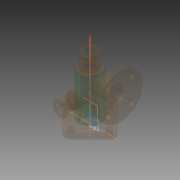
# Autodesk Inventor part: Piesa 3 3D
Saved by Autodesk Inventor 2011 SP2 (Build 150309200, 309)
## iProperties
Created: 2023-03-13
Part Number: Piesa 3 3D
Document SubType Name: Modeling
Designer: utilizator
Density: 1 g/cm^3
Author: utilizator
Autodesk Inventor part; units mm, degrees
ref_plane "XY Plane" through (0, 0, 0) normal (0, 0, 1) x (1, 0, 0)
sketch "Sketch1" plane through (0, 0, 0) normal (0, 0, 1) x (1, 0, 0)
  line L0 (-69.2965, 0) -> (69.2965, 0) projected
  line L1 (0, -69.2965) -> (0, 69.2965) projected
  line L2 (42.4264, -7.0711) -> (7.0711, -42.4264)
  line L3 (-7.0711, -42.4264) -> (-42.4264, -7.0711)
  line L4 (-42.4264, 7.0711) -> (-7.0711, 42.4264)
  line L5 (7.0711, 42.4264) -> (42.4264, 7.0711)
  arc A0 (7.0711, 42.4264) -> (-7.0711, 42.4264) centre (0, 35.3553) ccw
  arc A1 (42.4264, -7.0711) -> (42.4264, 7.0711) centre (35.3553, 0) ccw
  arc A2 (-7.0711, -42.4264) -> (7.0711, -42.4264) centre (0, -35.3553) ccw
  arc A3 (-42.4264, 7.0711) -> (-42.4264, -7.0711) centre (-35.3553, 0) ccw
  circle A4 centre (0, 35) radius 5
  circle A5 centre (35, 0) radius 5
  circle A6 centre (0, -35) radius 5
  circle A7 centre (-35, 0) radius 5
  point P0 (0, 0)
  point P1 (0, 0)
  point P2 (49.4975, 0)
  point P3 (0, -49.4975)
  point P4 (-49.4975, 0)
  point P5 (0, 49.4975)
  point P6 (0, 0)
  point P7 (0, 0)
  point P8 (0, -49.4975)
  point P9 (0, 0)
  point P10 (0, 0)
  point P11 (-49.4975, 0)
  point P12 (0, 0)
  point P13 (0, 0)
  point P14 (0, 49.4975)
  dimension "d0" = 70
  dimension "d1" = 10
  dimension "d2" = 10
  dimension "d3" = 10
  dimension "d4" = 10
  dimension "d5" = 5
  dimension "d6" = 35
  dimension "d9" = 360
  constraints: 10 point on line, 8 centre point, 8 end point, 8 point on circle, 8 tangent, 6 coincident, 1 vertical alignment, 27 other
  measures "d0" distance of point (0, 49.497) point (49.497, 0)
  measures "d1" radius of A0
  measures "d2" radius of A1
  measures "d3" radius of A2
  measures "d4" radius of A3
  measures "d5" radius of A4
  measures "d6" distance of point (0, 0) A4.centre
extrude "Extrusion1" add sketch "Sketch1" along normal blind 10 contours A3 L4 A0 L1 A4 L0 A7 | L0 A7 L1 A6 A2 L3 A3 | L1 A4 A0 L5 A1 L0 A5 | L0 A5 A1 L2 A2 L1 A6
sketch "Sketch2" plane through (0, 0, 10) normal (0, 0, 1) x (1, 0, 0)
  circle A0 centre (0, 0) radius 20
  dimension "d13" = 20
  constraints: 1 centre point, 1 coincident
  measures "d13" radius of A0
extrude "Extrusion2" add sketch "Sketch2" along normal blind 80 separate body
sketch "Sketch3" plane through (0, 0, 90) normal (0, 0, 1) x (1, 0, 0)
  circle A0 centre (0, 0) radius 20 projected
  circle A1 centre (0, 0) radius 15
  dimension "d16" = 15
  constraints: 1 centre point, 1 coincident
  measures "d16" radius of A1
extrude "Extrusion3" add sketch "Sketch3" along normal blind 25 separate body contours A1
ref_plane "Work Plane1" through (0, -55, 0) normal (0, 1, 0) x (-1, 0, 0)
sketch "Sketch4" plane through (0, -55, 0) normal (0, 1, 0) x (-1, 0, 0)
  circle A0 centre (0, 50) radius 13.5
  point P0 (0, 0)
  dimension "d20" = 13.5
  dimension "d21" = 50
  constraints: 1 centre point, 1 vertical alignment
  measures "d20" radius of A0
  measures "d21" distance of point (0, 0) A0.centre
extrude "Extrusion4" add sketch "Sketch4" along normal blind 24 separate body
sketch "Sketch5" plane through (0, -31, 50) normal (0, 1, 0) x (1, 0, 0)
  circle A0 centre (0, 0) radius 13.5 projected
  circle A1 centre (0, 0) radius 13
  point P0 (0, 50)
  dimension "d24" = 13
  constraints: 1 centre point, 1 coincident
  measures "d24" radius of A1
extrude "Extrusion5" add sketch "Sketch5" along normal blind 3 separate body contours A1
sketch "Sketch6" plane through (0, -28, 50) normal (0, 1, 0) x (1, 0, 0)
  circle A0 centre (0, 0) radius 13 projected
  circle A1 centre (0, 0) radius 15
  point P0 (0, 50)
  dimension "d27" = 15
  constraints: 1 centre point, 1 coincident
  measures "d27" radius of A1
extrude "Extrusion6" add sketch "Sketch6" along normal up to surface separate body contours A0 | A1 round surface about axis through (0, 0, 10) along (0, 0, 1) radius 20 far side no
ref_plane "Work Plane2" through (55, 0, 0) normal (1, 0, 0) x (0, 1, 0)
sketch "Sketch7" plane through (55, 0, 0) normal (1, 0, 0) x (0, 1, 0)
  circle A0 centre (0, 70) radius 40
  circle A1 centre (21.2132, 91.2132) radius 5
  circle A2 centre (21.2132, 48.7868) radius 5
  circle A3 centre (-21.2132, 48.7868) radius 5
  circle A4 centre (-21.2132, 91.2132) radius 5
  point P0 (0, 0)
  point P1 (25.813, 70)
  point P2 (0, 44.187)
  point P3 (-25.813, 70)
  point P4 (0, 95.813)
  dimension "d31" = 40
  dimension "d32" = 70
  dimension "d33" = 5
  dimension "d34" = 30
  dimension "d35" = 45
  dimension "d38" = 360
  constraints: 5 centre point, 2 coincident, 1 horizontal alignment, 1 vertical alignment, 14 other
  measures "d31" radius of A0
  measures "d32" distance of point (0, 0) A0.centre
  measures "d33" radius of A1
  measures "d34" distance of A0.centre A1.centre
extrude "Extrusion7" add sketch "Sketch7" against normal blind 10 separate body
sketch "Sketch8" plane through (45, 0, 70) normal (-1, 0, 0) x (0, 0, 1)
  circle A0 centre (0, 0) radius 40 projected
  circle A1 centre (0, 0) radius 15
  point P0 (-70, 0)
  dimension "d42" = 15
  constraints: 1 centre point, 1 coincident
  measures "d42" radius of A1
extrude "Extrusion8" add sketch "Sketch8" along normal up to surface separate body contours A1 round surface about axis through (0, 0, 10) along (0, 0, 1) radius 20 far side no
hole "Hole3" at (0, 0, 115) direction (0, 0, -1) diameter 16 depth 30 bodies 3 2
hole "Hole4" at (0, 0, 85) direction (0, 0, -1) diameter 25 depth 50 bodies 2
sketch "Sketch10" plane through (0, 0, 0) normal (0, 1, 0) x (-1, 0, 0)
  line L0 (0, -23) -> (0, 138) projected
  line L1 (12.5, 35) -> (-12.5, 35) projected
  line L2 (40, 0) -> (30, 0) projected
  line L3 (5, 0) -> (-5, 0) projected
  line L4 (-30, 0) -> (-40, 0) projected
  line L5 (5, 0) -> (-5, 0) projected
  line L6 (7.0711, 0) -> (42.4264, 0) projected
  line L7 (-7.0711, 0) -> (7.0711, 0) projected
  line L8 (-42.4264, 0) -> (-7.0711, 0) projected
  line L9 (-42.4264, 0) -> (-42.4264, 0) projected
  line L10 (-7.0711, 0) -> (-42.4264, 0) projected
  line L11 (7.0711, 0) -> (-7.0711, 0) projected
  line L12 (42.4264, 0) -> (7.0711, 0) projected
  line L13 (42.4264, 0) -> (42.4264, 0) projected
  line L14 (-12.5, 35) -> (-15, 0)
  line L15 (-15, 0) -> (0, 0)
  line L16 (0, 0) -> (0, 35)
  line L17 (-12.5, 35) -> (-15, 0)
  line L18 (0, 0) -> (0, 35)
  dimension "d82" = 15
  constraints: 10 end point, 3 collinear, 2 coincident, 1 midpoint, 1 point on line
  measures "d82" distance of L15.end L15.start
revolve "Revolution1" cut sketch "Sketch10" angle 360 about axis through (0, 0, -10) along (0, 0, 1) bodies 1
revolve "Revolution2" cut sketch "Sketch10" angle 360 about axis through (0, 0, -10) along (0, 0, 1) bodies 2
hole "Hole5" at (0, -55, 50) direction (0, 1, 0) diameter 15 depth 55 bodies 4
hole "Hole6" at (55, 0, 70) direction (-1, 0, 0) diameter 15 depth 55 bodies 7
chamfer "Chamfer1" distance 1 angle 45 3 edges at (-20, 0, 90) (-15, 0, 115) (13.5, -55, 50)
body "Solid1"
body "Solid2"
body "Solid3"
body "Solid4"
body "Solid5"
body "Solid6"
body "Solid7"
body "Solid8"
